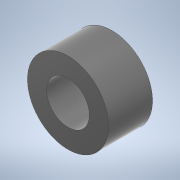
# Autodesk Inventor part: CCC-0612-65B
Saved by Autodesk Inventor 2022 (Build 260153000, 153)
## iProperties
Part Number: CCC-0612-65B
Material: アセタール樹脂、黒
Document SubType Name: Modeling
Designer: Masato Kubotera
Density: 1.07175 g/cm^3
Appearance: 滑らか - 黒
Mass: 0.57072 g
Surface Area: 5.37542 cm^2
Volume: 0.532512 cm^3
Description: CustomMade
Catalog Web Link: https://www.hirosugi-net.co.jp/shop/
Author: Masato Kubotera
Comments: CustomMade product The alternative is a combination of CC-0612-15B and CC-0612-50B.
Autodesk Inventor part; units mm, degrees
ref_plane "YZ Plane" through (0, 0, 0) normal (1, 0, 0) x (0, 1, 0)
ref_plane "XZ Plane" through (0, 0, 0) normal (0, 1, 0) x (-1, 0, 0)
ref_plane "XY Plane" through (0, 0, 0) normal (0, 0, 1) x (1, 0, 0)
sketch "スケッチ1" plane through (0, 0, 0) normal (0, 0, 1) x (1, 0, 0)
  circle A0 centre (0, 0) radius 3.15
  circle A1 centre (0, 0) radius 6
  dimension "d0" = 6.3
  dimension "d1" = 12
  constraints: 2 centre point, 2 coincident
  measures "d0" diameter of A0
  measures "d1" diameter of A1
extrude "押し出し1" add sketch "スケッチ1" along normal blind 6.5
